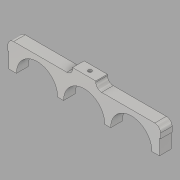
# Autodesk Inventor part: Tube Holder Halve 2
Saved by Autodesk Inventor 2017 (Build 210142000, 142)
## iProperties
Created: 2016-12-06
Part Number: Tube Holder Halve 2
Material: Aluminum 6061-AHC
Document SubType Name: Modeling
Designer: qupec
Density: 2.7 g/cm^3
Appearance: Aluminum - Dark
Mass: 20.4912 g
Surface Area: 43.8677 cm^2
Volume: 7.58934 cm^3
Author: qupec
Autodesk Inventor part; units mm, degrees
ref_plane "YZ Plane" through (0, 0, 0) normal (1, 0, 0) x (0, 1, 0)
ref_plane "XZ Plane" through (0, 0, 0) normal (0, 1, 0) x (-1, 0, 0)
ref_plane "XY Plane" through (0, 0, 0) normal (0, 0, 1) x (1, 0, 0)
sketch "Sketch1" plane through (0, 0, 0) normal (0, 0, 1) x (1, 0, 0)
  line L0 (-41.783, 14.2875) -> (41.783, 14.2875)
  line L1 (41.783, 14.2875) -> (41.783, -14.2875)
  line L2 (41.783, -14.2875) -> (-41.783, -14.2875)
  line L3 (-41.783, -14.2875) -> (-41.783, 14.2875)
  point P0 (0, 0)
  dimension "d0" = 83.566
  dimension "d1" = 41.783
  dimension "d2" = 14.2875
  dimension "d3" = 28.575
  constraints: 8 end point, 2 parallel, 1 horizontal, 1 perpendicular
  measures "d0" distance of L0.start L0.end
  measures "d1" distance from line of point (0, 0) L3
  measures "d2" distance from line of point (0, 0) L2
  measures "d3" distance of L2.end L0.start
extrude "Extrusion1" add sketch "Sketch1" along normal mid plane 6.35
sketch "Sketch2" plane through (0, 0, 3.175) normal (0, 0, 1) x (1, 0, 0)
  circle A0 centre (-25.781, 0) radius 11.303
  circle A1 centre (0, 0) radius 11.303
  line L0 (41.783, -14.2875) -> (41.783, 14.2875) projected
  circle A2 centre (25.781, 0) radius 11.303
  line L1 (-41.783, 14.2875) -> (-41.783, -14.2875) projected
  line L2 (-41.783, 0) -> (41.783, 0) construction
  line L3 (41.783, 14.2875) -> (-41.783, 14.2875) projected
  point P0 (0, 0)
  dimension "d6" = 22.606
  dimension "d9" = 22.606
  dimension "d11" = 22.606
  dimension "d14" = 25.781
  dimension "d21" = 83.566
  dimension "d22" = 25.781
  dimension "d45" = 0
  dimension "d88" = 3.175
  dimension "d89" = 3.175
  constraints: 3 centre point, 3 midpoint, 2 end point, 1 point on line
  measures "d6" diameter of A0
  measures "d9" diameter of A1
  measures "d11" diameter of A2
  measures "d14" distance of A1.centre A0.centre
  measures "d21" distance of L0.end L1.start
  measures "d22" distance of A2.centre A1.centre
  measures "d45" distance of point (0, 0) A1.centre
sketch "Sketch4" plane through (-41.783, -14.2875, -3.175) normal (-1, 0, 0) x (0, 0, 1)
  line L0 (0, 0) -> (0, 28.575) projected
  line L1 (6.35, 28.575) -> (6.35, 0) projected
  line L2 (0, 22.6695) -> (6.35, 22.6695)
  line L3 (6.35, 22.6695) -> (6.35, 5.9055)
  line L4 (6.35, 5.9055) -> (0, 5.9055)
  line L5 (0, 5.9055) -> (0, 22.6695)
  point P0 (3.175, 14.2875)
  dimension "d30" = 8.382
  dimension "d31" = 16.764
  constraints: 8 end point, 2 parallel, 1 horizontal, 1 perpendicular, 1 point on line, 2 other
  measures "d30" distance from line of point (3.175, 14.287) L4
  measures "d31" distance between parallel lines of L4 L2
extrude "Extrusion3" cut sketch "Sketch4" against normal blind 0.635
mirror "Mirror1" about plane through (0, 0, 0) normal (1, 0, 0) of "Extrusion3"
sketch "Sketch11" plane through (0, 0, -3.175) normal (0, 0, -1) x (-1, 0, 0)
  circle A0 centre (-37.211, 9.7155) radius 3.175
  line L0 (-41.783, 14.2875) -> (-41.783, 8.382) projected
  line L1 (41.783, 14.2875) -> (-41.783, 14.2875) projected
  point P0 (0, 0)
  dimension "d72" = 4.572
  dimension "d73" = 4.572
  dimension "d74" = 6.35
  constraints: 1 centre point
  measures "d72" distance from line of L0 A0.centre
  measures "d73" distance from line of L1 A0.centre
  measures "d74" diameter of A0
extrude "Extrusion10" cut sketch "Sketch11" against normal blind 1.27
sketch "Sketch7" plane through (-41.783, -14.2875, 3.175) normal (0, -1, 0) x (1, 0, 0)
  line L0 (27.813, -14.605) -> (55.753, -14.605)
  line L1 (55.753, -14.605) -> (55.753, 8.255)
  line L2 (55.753, 8.255) -> (27.813, 8.255)
  line L3 (27.813, 8.255) -> (27.813, -14.605)
  point P0 (41.783, -3.175)
  dimension "d39" = 27.94
  dimension "d40" = 22.86
  dimension "d41" = 11.43
  dimension "d42" = 13.97
  constraints: 8 end point, 2 parallel, 1 horizontal, 1 perpendicular
  measures "d39" distance of L0.start L0.end
  measures "d40" distance of L2.end L0.start
  measures "d41" distance from line of point (41.783, -3.175) L0
  measures "d42" distance from line of point (41.783, -3.175) L1
extrude "Extrusion5" [suppressed]
extrude "Extrusion6" cut sketch "Sketch2" against normal blind 25.4
sketch "Sketch8" plane through (0, 0, -3.175) normal (0, 0, -1) x (-1, 0, 0)
  line L0 (41.148, 8.382) -> (41.148, -8.382) construction
  line L1 (41.148, 0) -> (-41.148, 0)
  line L2 (-41.148, 8.382) -> (-41.148, -8.382) construction
  line L3 (41.783, 14.2875) -> (-41.783, 14.2875) projected
  line L4 (41.783, 8.382) -> (41.783, 14.2875) projected
  line L5 (-41.783, 14.2875) -> (-41.783, 8.382) projected
  line L6 (-41.148, 8.382) -> (-41.148, 0)
  line L7 (-41.783, 8.382) -> (-41.148, 8.382) projected
  line L8 (41.148, 8.382) -> (41.148, 0)
  line L9 (41.148, 8.382) -> (41.783, 8.382) projected
  point P0 (0, 0)
  constraints: 6 end point, 2 collinear, 2 midpoint
extrude "Extrusion7" [suppressed]
sketch "Sketch9" plane through (0, 0, -3.175) normal (0, 0, -1) x (-1, 0, 0)
  line L0 (-41.783, -14.2875) -> (41.783, -14.2875) projected
  line L1 (41.783, -14.2875) -> (41.783, -8.382) projected
  line L2 (41.783, -8.382) -> (41.148, -8.382) projected
  line L3 (-41.148, -8.382) -> (-41.783, -8.382) projected
  line L4 (-41.783, -8.382) -> (-41.783, -14.2875) projected
  line L5 (-41.148, 8.382) -> (-41.148, -8.382) projected
  line L6 (-41.148, 0) -> (-41.148, -8.382)
  line L7 (-41.148, 0) -> (41.148, 0)
  line L8 (41.148, -8.382) -> (41.148, 8.382) projected
  line L9 (41.148, -8.382) -> (41.148, 0)
  point P0 (0, 0)
  constraints: 6 end point, 2 collinear, 2 midpoint
extrude "Extrusion8" cut sketch "Sketch9" against normal through all
sketch "Sketch10" plane through (-41.148, 0, -3.175) normal (0, -1, 0) x (1, 0, 0)
  line L0 (4.064, 6.35) -> (4.064, 0) projected
  line L1 (0, 0) -> (0, 6.35) projected
  line L2 (-0.635, 0) -> (-0.635, 6.35) projected
  line L3 (4.064, 6.35) -> (4.064, 0) projected
  line L4 (0, 6.35) -> (4.064, 6.35) projected
  line L5 (0, 0) -> (0, 6.35) projected
  line L6 (4.064, 0) -> (0, 0) projected
  circle A0 centre (2.032, 3.81) radius 1.5494
  line L7 (81.534, 1.27) -> (75.184, 1.27) projected
  line L8 (81.534, 0) -> (75.184, 0) projected
  point P0 (41.148, 3.175)
  point P1 (84.328, 1.27)
  point P2 (77.978, 1.27)
  point P3 (84.328, 0)
  point P4 (77.978, 0)
  dimension "d58" = 3.0988
  dimension "d61" = 4.064
  dimension "d62" = 2.032
  dimension "d77" = 5.08
  dimension "d78" = 2.54
  constraints: 1 centre point
  measures "d58" diameter of A0
  measures "d61" distance of L3.end L5.start
  measures "d62" distance from line of A0.centre L1
  measures "d77" distance between parallel lines of L4 L7
  measures "d78" distance from line of L4 A0.centre
extrude "Extrusion9" cut sketch "Sketch10" against normal blind 11.43 contours A0
mirror "Mirror2" about plane through (0, 0, 0) normal (1, 0, 0) of "Extrusion9"
thread "Thread1" size "5-40 UNC" class "2B" standard "ANSI Unified Screw Threads" full length
thread "Thread2" size "5-40 UNC" class "2B" standard "ANSI Unified Screw Threads" full length
fillet "Fillet1" radius 3.175 2 edges at (-41.783, 14.2875, 0) (41.783, 14.2875, 0)
sketch "Sketch12" plane through (-38.608, 14.2875, -3.175) normal (0, 1, 0) x (1, 0, 0)
  line L0 (77.216, -6.35) -> (0, -6.35) projected
  line L1 (32.258, 0) -> (44.958, 0)
  line L2 (44.958, 0) -> (44.958, -6.35)
  line L3 (44.958, -6.35) -> (32.258, -6.35)
  line L4 (32.258, -6.35) -> (32.258, 0)
  circle A0 centre (38.608, -3.175) radius 1
  line L5 (27.305, 0) -> (49.911, 0) projected
  dimension "d81" = 6.35
  dimension "d82" = 12.7
  dimension "d83" = 2
  dimension "d87" = 0
  constraints: 8 end point, 2 parallel, 1 centre point, 1 coincident, 1 horizontal, 1 perpendicular, 1 point on line
  measures "d81" distance from line of point (38.608, -3.175) L4
  measures "d82" distance of L1.start L1.end
  measures "d83" diameter of A0
  measures "d87" distance between parallel lines of L5 L1
extrude "Extrusion11" add sketch "Sketch12" along normal blind 3.8
fillet "Fillet3" radius 3.175 2 edges at (6.35, 14.2875, 0) (-6.35, 14.2875, 0)
equation "\"d1\" = 0.5 * d0"
equation "\"d2\" = 0.5 * d3"
equation "\"d9\" = d7"
equation "\"d11\" = d9"
equation "\"d22\" = d14"
equation "\"d30\" = 0.5 * d31"
equation "\"d41\" = 0.5 * d40"
equation "\"d42\" = 0.5 * d39"
equation "\"d62\" = 0.5 * d61"
equation "\"d78\" = 0.5 * d77"
equation "\"d81\" = 0.5 * d82"
equation "\"d7\" = d6"
body "Solid1"
